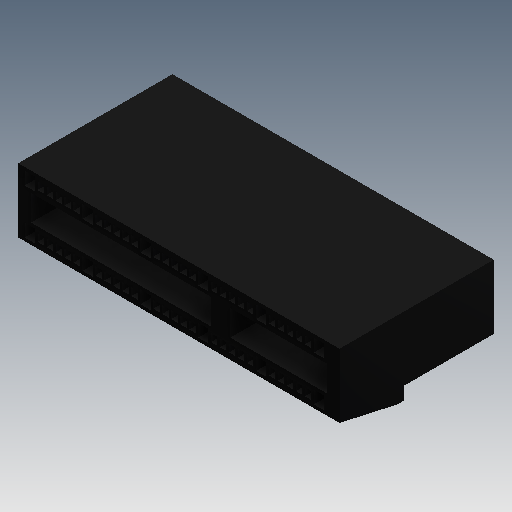
# Autodesk Inventor part: config - pcie connector
Saved by Autodesk Inventor 2019.1 (Build 231200000, 200)
## iProperties
Company: Autodesk Asia Pte. Ltd.
Created: 2005-12-05
Part Number: config - pcie connector
Document SubType Name: Modeling
Designer: Simon.Ng@autodesk.com
Stock Number: config - pcie connector
Density: 1 g/cm^3
Material: Generic
Mass: 1.09695 g
Surface Area: 21.9884 cm^2
Volume: 1.09695 cm^3
Appearance: Glossy - Black
Title: PC Demo
Author: Simon.Ng@autodesk.com
Autodesk Inventor part; units mm, degrees
ref_plane "YZ Plane" through (0, 0, 0) normal (1, 0, 0) x (0, 1, 0)
ref_plane "XZ Plane" through (0, 0, 0) normal (0, 1, 0) x (-1, 0, 0)
ref_plane "XY Plane" through (0, 0, 0) normal (0, 0, 1) x (1, 0, 0)
sketch "Sketch1" plane through (0, 0, 0) normal (0, 0, 1) x (1, 0, 0)
  line L0 (0, 4) -> (0, -3) construction
  line L1 (-15, 0) -> (20, 0) construction
  line L2 (-12.5, 2.5) -> (12.5, 2.5)
  line L3 (12.5, 2.5) -> (12.5, -2.5)
  line L4 (12.5, -2.5) -> (-12.5, -2.5)
  line L5 (-12.5, -2.5) -> (-12.5, 2.5)
  dimension "d0" = 25
  dimension "d1" = 5
  constraints: 8 end point, 2 parallel, 1 horizontal, 1 perpendicular, 2 other
  measures "d0" distance of L2.start L2.end
  measures "d1" distance of L4.end L2.start
extrude "Extrusion1" add sketch "Sketch1" along normal blind 12
sketch "Sketch2" plane through (0, 0, 12) normal (0, 0, 1) x (1, 0, 0)
  line L0 (12.5, 2.5) -> (12.5, -2.5) projected
  line L1 (-12.5, -2.5) -> (-12.5, 2.5) projected
  line L2 (-12.5, 0) -> (12.5, 0) construction
  line L3 (-11.5, 1) -> (2.5, 1)
  line L4 (2.5, 1) -> (2.5, -1)
  line L5 (2.5, -1) -> (-11.5, -1)
  line L6 (-11.5, -1) -> (-11.5, 1)
  line L7 (4, 1) -> (11.5, 1)
  line L8 (11.5, 1) -> (11.5, -1)
  line L9 (11.5, -1) -> (4, -1)
  line L10 (4, -1) -> (4, 1)
  dimension "d4" = 1
  dimension "d5" = 2
  dimension "d6" = 14
  dimension "d7" = 1.5
  dimension "d8" = 1
  dimension "d9" = 7.5
  constraints: 18 end point, 4 parallel, 2 horizontal, 2 midpoint, 2 perpendicular, 1 collinear, 2 other
  measures "d4" distance between parallel lines of L1 L6
  measures "d5" distance of L5.end L3.start
  measures "d6" distance of L3.start L3.end
  measures "d7" distance between parallel lines of L10 L4
  measures "d8" distance between parallel lines of L0 L8
  measures "d9" distance of L7.start L7.end
extrude "Extrusion2" cut sketch "Sketch2" against normal blind 8
sketch "Sketch3" plane through (0, 0, 12) normal (0, 0, 1) x (1, 0, 0)
  line L0 (-11.5, 1) -> (2.5, 1) projected
  line L1 (-12.5, 2.5) -> (12.5, 2.5) projected
  line L2 (-12.5, -2.5) -> (-12.5, 2.5) projected
  line L3 (-27.2504, 2.5) -> (-27.2504, 1) construction
  line L4 (-27.2504, 1.75) -> (-12.5, 1.75) construction
  line L5 (-12, 2.25) -> (-11.2, 2.25)
  line L6 (-11.2, 2.25) -> (-11.2, 1.25)
  line L7 (-11.2, 1.25) -> (-12, 1.25)
  line L8 (-12, 1.25) -> (-12, 2.25)
  line L9 (-11, 2.05) -> (-10.5, 2.05)
  line L10 (-10.5, 2.05) -> (-10.5, 1.45)
  line L11 (-10.5, 1.45) -> (-11, 1.45)
  line L12 (-11, 1.45) -> (-11, 2.05)
  line L13 (-10.3, 2.05) -> (-9.8, 2.05)
  line L14 (-9.8, 2.05) -> (-9.8, 1.45)
  line L15 (-9.8, 1.45) -> (-10.3, 1.45)
  line L16 (-10.3, 1.45) -> (-10.3, 2.05)
  line L17 (-9.6, 2.05) -> (-9.1, 2.05)
  line L18 (-9.1, 2.05) -> (-9.1, 1.45)
  line L19 (-9.1, 1.45) -> (-9.6, 1.45)
  line L20 (-9.6, 1.45) -> (-9.6, 2.05)
  line L21 (-8.9, 2.05) -> (-8.4, 2.05)
  line L22 (-8.4, 2.05) -> (-8.4, 1.45)
  line L23 (-8.4, 1.45) -> (-8.9, 1.45)
  line L24 (-8.9, 1.45) -> (-8.9, 2.05)
  line L25 (-8.2, 2.05) -> (-7.7, 2.05)
  line L26 (-7.7, 2.05) -> (-7.7, 1.45)
  line L27 (-7.7, 1.45) -> (-8.2, 1.45)
  line L28 (-8.2, 1.45) -> (-8.2, 2.05)
  dimension "d12" = 0.8
  dimension "d13" = 1
  dimension "d14" = 0.2
  dimension "d15" = 0.5
  dimension "d16" = 0.5
  dimension "d17" = 0.6
  dimension "d20" = 0.7
  constraints: 52 end point, 4 parallel, 4 perpendicular, 3 horizontal, 3 point on line, 1 midpoint, 34 other
  measures "d12" distance of L5.start L5.end
  measures "d13" distance of L7.end L5.start
  measures "d14" distance between parallel lines of L6 L12
  measures "d15" distance between parallel lines of L2 L8
  measures "d16" distance of L9.start L9.end
  measures "d17" distance of L9.end L10.end
  measures "d20" distance of L9.start L13.start
extrude "Extrusion3" cut sketch "Sketch3" against normal blind 5
pattern_linear "Rectangular Pattern1" count 5 spacing 4.5 along (1, 0, 0) of "Extrusion3"
sketch "Sketch5" plane through (0, 0, 12) normal (0, 0, 1) x (1, 0, 0)
  line L0 (10.3, 2.05) -> (10.3, 1.45) projected
  line L1 (6, 2.25) -> (6.8, 2.25) projected
  line L2 (6.8, 1.25) -> (6, 1.25) projected
  line L3 (10.5, 2.25) -> (11.3, 2.25)
  line L4 (11.3, 2.25) -> (11.3, 1.25)
  line L5 (11.3, 1.25) -> (10.5, 1.25)
  line L6 (10.5, 1.25) -> (10.5, 2.25)
  dimension "d37" = 0.2
  dimension "d38" = 0.8
  constraints: 8 end point, 2 collinear, 2 parallel, 1 horizontal, 1 perpendicular
  measures "d37" distance between parallel lines of L6 L0
  measures "d38" distance of L3.start L3.end
extrude "Extrusion5" cut sketch "Sketch5" against normal blind 8
mirror "Mirror2" about plane through (0, 0, 0) normal (0, 1, 0) of "Extrusion3", "Rectangular Pattern1", "Extrusion5"
sketch "Sketch6" plane through (12.5, -2.5, 0) normal (1, 0, 0) x (0, 0, -1)
  line L0 (0, 0) -> (-12, 0) projected
  line L1 (0, 5) -> (-12, 5) projected
  line L2 (-12, 0) -> (-7.5, -1)
  line L3 (-7.5, -1) -> (-7, -1)
  line L4 (-7, -1) -> (-7, 0)
  dimension "d41" = 1
  dimension "d42" = 4.5
  dimension "d43" = 0.5
  constraints: 6 end point, 1 parallel, 1 perpendicular, 1 point on line
  measures "d41" distance between parallel lines of L3 L0
  measures "d42" horizontal distance of L0.end L2.end
  measures "d43" distance of L2.end L3.end
extrude "Extrusion6" add sketch "Sketch6" against normal up to surface (25 mm away)
body "Solid1"
